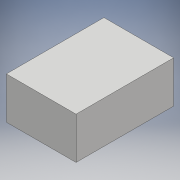
# Autodesk Inventor part: Pièce_roue folle
Saved by Autodesk Inventor 2017.3 (Build 213256000, 256)
## iProperties
Part Number: Pièce_roue folle
Material: Générique
Document SubType Name: Modeling
Designer: Piou piou
Density: 1 g/cm^3
Appearance: Par défaut
Author: Piou piou
Autodesk Inventor part; units mm, degrees
ref_plane "YZ Plane" through (0, 0, 0) normal (1, 0, 0) x (0, 1, 0)
ref_plane "XZ Plane" through (0, 0, 0) normal (0, 1, 0) x (-1, 0, 0)
ref_plane "XY Plane" through (0, 0, 0) normal (0, 0, 1) x (1, 0, 0)
sketch "Esquisse1" plane through (0, 0, 0) normal (0, 1, 0) x (-1, 0, 0)
  line L0 (-25, 15) -> (25, 15)
  line L1 (25, 15) -> (25, -15)
  line L2 (25, -15) -> (-25, -15)
  line L3 (-25, -15) -> (-25, 15)
  line L4 (-25, 15) -> (25, -15) construction
  line L5 (25, 15) -> (-25, -15) construction
  line L6 (-22, 12) -> (22, 12)
  line L7 (22, 12) -> (22, -12)
  line L8 (22, -12) -> (-22, -12)
  line L9 (-22, -12) -> (-22, 12)
  line L10 (-22, 12) -> (22, -12) construction
  line L11 (22, 12) -> (-22, -12) construction
  point P0 (0, 0)
  dimension "d0" = 50
  dimension "d1" = 30
  dimension "d2" = 3
  dimension "d3" = 3
  constraints: 24 end point, 4 midpoint, 4 parallel, 2 horizontal, 2 perpendicular
  measures "d0" distance of L1.end L2.end
  measures "d1" distance of L0.end L1.end
  measures "d2" distance between parallel lines of L2 L8
  measures "d3" distance between parallel lines of L1 L7
extrude "Extrusion1" add sketch "Esquisse1" along normal blind 5 contours L0 L1 L2 L3 | L6 L7 L8 L9
sketch "Esquisse2" plane through (0, 0, 0) normal (0, -1, 0) x (1, 0, 0)
  line L0 (-22, 12) -> (22, 12)
  line L1 (22, 12) -> (22, -12)
  line L2 (22, -12) -> (-22, -12)
  line L3 (-22, -12) -> (-22, 12)
  line L4 (-22, 12) -> (22, -12) construction
  line L5 (22, 12) -> (-22, -12) construction
  line L6 (-25, -15) -> (25, -15) projected
  line L7 (25, -15) -> (25, 15) projected
  line L8 (25, 15) -> (-25, 15) projected
  line L9 (-25, 15) -> (-25, -15) projected
  point P0 (0, 0)
  dimension "d6" = 3
  dimension "d7" = 3
  constraints: 12 end point, 2 midpoint, 2 parallel, 1 horizontal, 1 perpendicular
  measures "d6" distance between parallel lines of L6 L2
  measures "d7" distance between parallel lines of L7 L1
extrude "Extrusion2" add sketch "Esquisse2" along normal blind 60
sketch "Esquisse3" plane through (0, -60, 0) normal (0, -1, 0) x (1, 0, 0)
  line L0 (25, -15) -> (25, 15) projected
  line L1 (-25, -15) -> (25, -15) projected
  line L2 (25, 15) -> (-25, 15) projected
  line L3 (-25, 15) -> (-25, -15) projected
  point P0 (0, 0)
extrude "Extrusion3" add sketch "Esquisse3" along normal blind 5
sketch "Esquisse4" plane through (0, 5, 0) normal (0, 1, 0) x (1, 0, 0)
  point P0 (0, 0)
